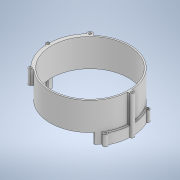
# Autodesk Inventor part: NewShooterCup
Saved by Autodesk Inventor 2020 (Build 240168000, 168)
## iProperties
Created: 2021-04-21
Part Number: NewShooterCup
Material: Generic
Document SubType Name: Modeling
Designer: tdmp4
Density: 1 g/cm^3
Appearance: Default
Author: tdmp4
Autodesk Inventor part; units mm, degrees
ref_plane "YZ Plane" through (0, 0, 0) normal (1, 0, 0) x (0, 1, 0)
ref_plane "XZ Plane" through (0, 0, 0) normal (0, 1, 0) x (-1, 0, 0)
ref_plane "XY Plane" through (0, 0, 0) normal (0, 0, 1) x (1, 0, 0)
sketch "Sketch1" plane through (0, 0, 0) normal (0, 1, 0) x (-1, 0, 0)
  circle A0 centre (0, 0) radius 72.39
  circle A1 centre (0, 0) radius 69.85
  arc A2 (-76.197, 3.807) -> (-76.197, -3.807) centre (-76.197, 0) ccw
  circle A3 centre (-76.197, 0) radius 2.286
  line L0 (-76.197, 3.807) -> (-72.2898, 3.807)
  line L1 (-76.197, -3.807) -> (-72.2898, -3.807)
  dimension "d0" = 144.78
  dimension "d1" = 139.7
  dimension "d2" = 4.572
  constraints: 4 centre point, 4 end point, 4 point on circle, 3 coincident, 1 horizontal, 1 tangent
  measures "d0" diameter of A0
  measures "d1" diameter of A1
  measures "d2" diameter of A3
extrude "Extrusion1" add sketch "Sketch1" along normal blind 50.8
sketch "Sketch2" plane through (0, 50.8, 0) normal (0, 1, 0) x (1, 0, 0)
  circle A0 centre (76.197, 0) radius 2.286 projected
  circle A1 centre (0, 0) radius 76.197
  arc A2 (-76.1019, 3.8058) -> (-76.1019, -3.8058) centre (-76.197, 0) ccw
  arc A3 (72.2898, 3.807) -> (72.2898, -3.807) centre (0, 0) ccw projected
  arc A4 (-76.1627, 2.2857) -> (-76.1627, -2.2857) centre (-76.197, 0) ccw
  line L0 (-76.197, -3.807) -> (-72.2898, -3.807)
  line L1 (-76.197, 3.807) -> (-72.39, 3.807)
  line L2 (-51.1875, 51.1875) -> (-53.8794, 53.8794)
  line L3 (0, 0) -> (76.197, 0) construction
  line L4 (0, 0) -> (76.197, 0) construction
  arc A5 (-56.5033, -51.1211) -> (-50.7603, -56.0621) centre (-53.8794, -53.8794) ccw
  line L5 (-51.1211, -56.5033) -> (-48.7078, -53.5524)
  line L6 (-56.5033, -51.1211) -> (-53.744, -48.4963)
  circle A6 centre (-53.8794, -53.8794) radius 2.286
  circle A7 centre (-53.8794, 53.8794) radius 2.286
  line L7 (-57.0474, 50.5132) -> (-54.2736, 47.9029)
  line L8 (-50.5132, 57.0474) -> (-47.9029, 54.2736)
  arc A8 (-50.5132, 57.0474) -> (-57.0474, 50.5132) centre (-53.8794, 53.8794) ccw
  line L9 (0, 0) -> (-26.9652, -26.9652)
  circle A9 centre (-76.197, 0) radius 2.286
  point P0 (-76.1627, -2.2857)
  dimension "d5" = 4.572
  dimension "d6" = 135
  dimension "d8" = 4.572
  dimension "d9" = 4.572
  constraints: 20 end point, 17 point on circle, 6 centre point, 6 coincident, 6 tangent, 3 horizontal, 2 point on line, 1 parallel, 16 other
  measures "d5" diameter of A4
  measures "d6" angle of L3 L2
  measures "d8" diameter of A6
  measures "d9" diameter of A7
extrude "Extrusion2" add sketch "Sketch2" against normal blind 25.4 contours L8 A3 L2 A7 A1 | A1 A7 A8 | A5 A1 A6 | A1 A6 L6 A3 L5 | L7 A3 L0 A1 A9 | A1 A7 L2 A3 L7 | A1 L0 A3 L6 | A1 A4 A2
sketch "Sketch3" plane through (0, 0, 0) normal (0, -1, 0) x (1, 0, 0)
  line L0 (72.2898, 3.807) -> (76.197, 3.807) projected
  circle A0 centre (0, 0) radius 72.39
  circle A1 centre (0, 0) radius 69.85
  line L1 (-69.85, 0) -> (52.6357, 45.9184)
  circle A2 centre (0, 0) radius 69.85 projected
  line L2 (-69.85, 0) -> (52.6357, -45.9184)
  line L3 (52.6357, 45.9184) -> (55.1695, 46.8683)
  arc A3 (72.2898, 3.807) -> (-48.7078, 53.5524) centre (0, 0) ccw projected
  line L4 (52.6357, -45.9184) -> (55.1695, -46.8683)
  dimension "d12" = 130.81
  constraints: 8 end point, 5 point on circle, 2 coincident, 1 centre point, 3 other
  measures "d12" distance of L1.start L1.end
extrude "Extrusion3" add sketch "Sketch3" along normal blind 19.05 contours A0 L4 A1 L3 picked at (58.6234, 40.6965)
sketch "Sketch4" plane through (0, 0, 0) normal (0, -1, 0) x (1, 0, 0)
  circle A0 centre (76.197, 0) radius 2.286 projected
  circle A1 centre (76.197, 0) radius 2.286
  arc A2 (76.197, -3.807) -> (76.197, 3.807) centre (76.197, 0) ccw
  line L0 (76.197, -3.807) -> (72.2898, -3.807) projected
  line L1 (76.197, -3.807) -> (72.2898, -3.807)
  line L2 (72.2898, 3.807) -> (76.197, 3.807) projected
  line L3 (76.197, 3.807) -> (72.2898, 3.807)
  arc A3 (72.2898, -3.807) -> (72.2898, 3.807) centre (0, 0) ccw projected
  line L4 (72.2898, 3.807) -> (72.2898, -3.807)
  circle A4 centre (0, 0) radius 76.197
  line L5 (0, 0) -> (76.197, 0) construction
  line L6 (0, 0) -> (76.197, 0) construction
  arc A5 (67.8091, 34.755) -> (64.0033, 41.3469) centre (65.9886, 38.0985) ccw
  arc A6 (64.0033, -41.3469) -> (67.8091, -34.755) centre (65.9886, -38.0985) ccw
  circle A7 centre (65.9886, -38.0985) radius 2.286
  circle A8 centre (65.9886, 38.0985) radius 2.286
  line L7 (64.0033, 41.3469) -> (60.7024, 39.4402)
  line L8 (67.8091, 34.755) -> (64.4936, 32.8768)
  arc A9 (55.1695, -46.8683) -> (55.1695, 46.8683) centre (0, 0) ccw projected
  line L9 (67.8105, -34.7524) -> (64.4936, -32.8768)
  line L10 (64.0017, -41.3494) -> (60.6368, -39.541)
  line L11 (64.0088, 36.9555) -> (65.9886, 38.0985)
  line L12 (62.689, -36.1935) -> (62.6916, -36.195)
  line L13 (64.0088, -36.9555) -> (65.9886, -38.0985)
  arc A10 (62.7648, -36.068) -> (62.6181, -36.3219) centre (65.9886, -38.0985) ccw
  arc A11 (64.0017, -41.3494) -> (67.8105, -34.7524) centre (65.9886, -38.0985) ccw
  point P0 (76.1019, -3.807)
  point P1 (76.1019, 3.807)
  dimension "d18" = 4.572
  dimension "d19" = 4.572
  constraints: 24 end point, 11 point on circle, 8 coincident, 6 centre point, 4 horizontal, 1 perpendicular, 1 point on line, 24 other
extrude "Extrusion4" add sketch "Sketch4" along normal blind 19.05 contours A0 A4 L2 A2 L0 | A0 A4 L0 A3 L2 | L2 A9 L8 A4 | A4 L9 A9 L0 | L8 A9 L7 A4 A8 | A4 A8 A5 | A11 A4 A6 | A4 A7 L10 A9 L9 | A6 A4 A7
sketch "Sketch5" plane through (0, 25.4, 0) normal (0, -1, 0) x (1, 0, 0)
  circle A0 centre (-76.197, 0) radius 2.286 projected
  circle A1 centre (-76.197, 0) radius 2.286
  arc A2 (-76.1019, 3.8058) -> (-76.1019, -3.8058) centre (-76.197, 0) ccw
  arc A3 (-76.1019, -3.8058) -> (-57.0474, -50.5132) centre (0, 0) ccw projected
  line L0 (-76.1019, -3.8058) -> (-72.2948, -3.7107)
  arc A4 (-48.7078, 53.5524) -> (-47.9029, -54.2736) centre (0, 0) ccw projected
  arc A5 (-56.5033, 51.1211) -> (-76.1019, 3.8058) centre (0, 0) ccw projected
  line L1 (-76.1019, 3.8058) -> (-72.2948, 3.8058)
  line L2 (-72.2948, -3.7107) -> (-72.2948, 3.8058)
  point P0 (-72.2948, 3.7107)
  constraints: 6 end point, 4 point on circle, 2 centre point, 2 coincident, 1 horizontal, 1 point on line, 1 vertical
extrude "Extrusion5" add sketch "Sketch5" along normal blind 44.45 contours L1 L2 A4 L0 A2
body "Solid1"
